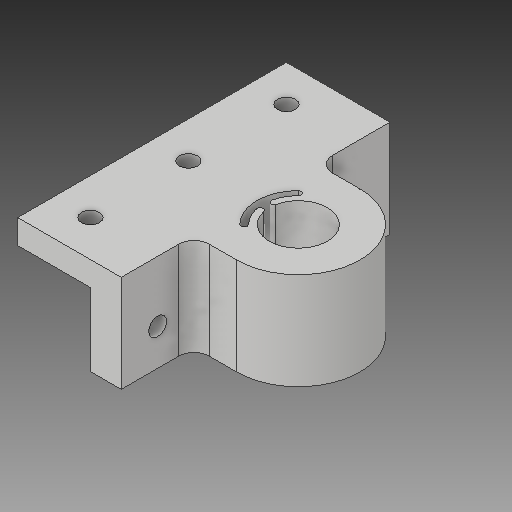
# Autodesk Inventor part: AxleBracket(3)
Saved by Autodesk Inventor 2018 (Build 220112000, 112)
## iProperties
Created: 2019-02-17
Part Number: AxleBracket(3)
Material: Generic
Document SubType Name: Modeling
Designer: anirudh
Density: 1 g/cm^3
Appearance: Default
Mass: 17.8737 g
Surface Area: 77.8022 cm^2
Volume: 17.8737 cm^3
Author: anirudh
Autodesk Inventor part; units mm, degrees
ref_plane "YZ Plane" through (0, 0, 0) normal (1, 0, 0) x (0, 1, 0)
ref_plane "XZ Plane" through (0, 0, 0) normal (0, 1, 0) x (-1, 0, 0)
ref_plane "XY Plane" through (0, 0, 0) normal (0, 0, 1) x (1, 0, 0)
sketch "Sketch1" plane through (0, 0, 0) normal (0, 1, 0) x (-1, 0, 0)
  arc A0 (0, 12.7) -> (0, -12.7) centre (0, 0) ccw
  line L0 (15.1638, 0) -> (15.1638, 12.7)
  line L1 (15.1638, 12.7) -> (15.1638, -12.7)
  line L2 (0, 12.7) -> (15.1638, 12.7)
  line L3 (0, -12.7) -> (15.1638, -12.7)
  arc A1 (6.0347, -6.0347) -> (6.0347, 6.0347) centre (0, 0) ccw
  arc A2 (5.8608, 1.285) -> (5.8669, -1.2566) centre (0, 0) ccw
  arc A3 (5.8608, 1.285) -> (5.8669, -1.2566) centre (0, 0) ccw
  arc A4 (5.8608, 1.285) -> (7.0867, 1.5971) centre (6.4884, 1.3835) ccw
  arc A5 (5.8608, 1.285) -> (7.0867, 1.5971) centre (6.4884, 1.3835) ccw
  arc A6 (7.0867, 1.5971) -> (5.1367, 5.1367) centre (0, 0) ccw
  arc A7 (6.0347, 6.0347) -> (5.1367, 5.1367) centre (5.5857, 5.5857) ccw
  arc A8 (6.0347, 6.0347) -> (5.1367, 5.1367) centre (5.5857, 5.5857) ccw
  arc A9 (5.1367, -5.1367) -> (6.0347, -6.0347) centre (5.5857, -5.5857) ccw
  arc A10 (5.1367, -5.1367) -> (6.0347, -6.0347) centre (5.5857, -5.5857) ccw
  arc A11 (7.0897, -1.5835) -> (5.8669, -1.2566) centre (6.4591, -1.4921) ccw
  arc A12 (7.0659, -1.6865) -> (5.8237, -1.444) centre (6.4591, -1.4921) ccw
  arc A13 (5.1367, -5.1367) -> (7.0897, -1.5835) centre (0, 0) ccw
  constraints: 36 point on circle, 14 centre point, 8 coincident, 8 end point, 2 perpendicular, 1 tangent
extrude "Extrusion1" add sketch "Sketch1" along normal blind 15
sketch "Sketch2" plane through (-15.1638, 0, 12.7) normal (0, 0, 1) x (1, 0, 0)
  line L0 (0, 15) -> (15.1638, 15) projected
  line L1 (15.1638, 0) -> (0, 0) projected
  line L2 (0, 15) -> (6.35, 15)
  line L3 (6.35, 15) -> (6.35, 0)
  line L4 (6.35, 0) -> (0, 0)
  line L5 (0, 0) -> (0, 15)
  dimension "d5" = 6.35
  constraints: 8 end point, 2 parallel, 1 horizontal, 1 perpendicular, 1 point on line
  measures "d5" distance of L3.end L4.end
extrude "Extrusion2" add sketch "Sketch2" along normal blind 15
sketch "Sketch3" plane through (0, 0, -12.7) normal (0, 0, -1) x (-1, 0, 0)
  line L0 (0, 15) -> (15.1638, 15) projected
  line L1 (15.1638, 0) -> (0, 0) projected
  line L2 (15.1638, 15) -> (8.8138, 15)
  line L3 (8.8138, 15) -> (8.8138, 0)
  line L4 (8.8138, 0) -> (15.1638, 0)
  line L5 (15.1638, 0) -> (15.1638, 15)
  dimension "d8" = 6.35
  constraints: 8 end point, 2 parallel, 1 horizontal, 1 perpendicular, 1 point on line
  measures "d8" distance of L4.end L3.end
extrude "Extrusion3" add sketch "Sketch3" along normal blind 15
sketch "Sketch4" plane through (-8.8138, 0, 12.7) normal (1, 0, 0) x (0, 0, -1)
  line L0 (-15, 15) -> (40.4, 15) projected
  line L1 (0, 0) -> (0, 15) projected
  line L2 (25.4, 15) -> (40.4, 15) projected
  line L3 (25.4, 0) -> (40.4, 0) projected
  line L4 (40.4, 0) -> (40.4, 15) projected
  line L5 (25.4, 0) -> (25.4, 15) projected
  circle A0 centre (-7.5, 7.5) radius 1.85
  circle A1 centre (32.9, 7.5) radius 1.85
  point P0 (12.7, 0)
  point P1 (-15, 0)
  dimension "d13" = 3.7
  dimension "d14" = 3.7
  constraints: 2 centre point
  measures "d13" diameter of A0
  measures "d14" diameter of A1
extrude "Extrusion4" cut sketch "Sketch4" against normal blind 15 contours A0 | A1
sketch "Sketch5" plane through (0, 15, 0) normal (0, 1, 0) x (1, 0, 0)
  line L0 (-8.8138, 12.7) -> (-8.8138, 27.7) projected
  line L1 (-15.1638, -27.7) -> (-8.8138, -27.7)
  line L2 (-8.8138, 27.7) -> (-15.1638, 27.7)
  line L3 (-8.8138, -12.7) -> (-8.8138, -27.7) projected
  line L4 (-8.8138, -27.7) -> (-8.8138, -12.7)
  arc A0 (0, -12.7) -> (0, 12.7) centre (0, 0) ccw projected
  line L5 (-8.8138, -12.7) -> (0, -12.7)
  line L6 (-8.8138, 27.7) -> (-8.8138, 12.7)
  line L7 (0, 12.7) -> (-8.8138, 12.7) projected
  line L8 (-8.8138, 12.7) -> (0, 12.7)
  arc A1 (0, -12.7) -> (0, 12.7) centre (0, 0) ccw
  arc A2 (-5.8752, -1.2175) -> (-5.8669, 1.2566) centre (0, 0) ccw
  arc A3 (-6.0347, -6.0347) -> (-5.1367, -5.1367) centre (-5.5857, -5.5857) ccw projected
  arc A4 (-6.0347, -6.0347) -> (-5.1367, -5.1367) centre (-5.5857, -5.5857) ccw
  arc A5 (-5.8608, -1.285) -> (-7.0867, -1.5971) centre (-6.4884, -1.3835) ccw projected
  arc A6 (-5.8608, -1.285) -> (-7.0867, -1.5971) centre (-6.4884, -1.3835) ccw
  arc A7 (-7.0897, 1.5835) -> (-5.8669, 1.2566) centre (-6.4591, 1.4921) ccw projected
  arc A8 (-7.0659, 1.6865) -> (-5.8237, 1.444) centre (-6.4591, 1.4921) ccw
  arc A9 (-5.1367, 5.1367) -> (-6.0347, 6.0347) centre (-5.5857, 5.5857) ccw projected
  arc A10 (-5.1367, 5.1367) -> (-6.0347, 6.0347) centre (-5.5857, 5.5857) ccw
  arc A11 (-7.0867, -1.5971) -> (-5.1367, -5.1367) centre (0, 0) ccw projected
  arc A12 (-6.0347, 6.0347) -> (-6.0347, -6.0347) centre (0, 0) ccw
  arc A13 (-5.1367, 5.1367) -> (-7.0897, 1.5835) centre (0, 0) ccw
  arc A14 (-7.1217, -1.4326) -> (-5.1367, -5.1367) centre (0, 0) ccw
  line L9 (-15.1638, -27.7) -> (-30.1638, -27.7)
  line L10 (-30.1638, -27.7) -> (-30.1638, 27.7)
  line L11 (-30.1638, 27.7) -> (-15.1638, 27.7)
  circle A15 centre (-22.6638, -20.2) radius 1.85
  circle A16 centre (-22.6638, 0) radius 1.85
  circle A17 centre (-22.6638, 20.2) radius 1.85
  dimension "d17" = 15
  dimension "d18" = 3.7
  dimension "d19" = 3.7
  dimension "d20" = 3.7
  constraints: 28 point on circle, 18 end point, 12 centre point, 8 coincident, 3 equal length, 3 perpendicular, 2 horizontal, 1 tangent, 1 vertical
  measures "d17" distance of L1.start L9.end
  measures "d18" diameter of A15
  measures "d19" diameter of A16
  measures "d20" diameter of A17
extrude "Extrusion5" add sketch "Sketch5" along normal blind 5 contours L7 A0 L5 L3 L1 L9 L10 L11 L2 L0 | A14 A5
fillet "Fillet1" radius 3.175 2 edges at (-8.8138, 10, 12.7) (-8.8138, 10, -12.7)
body "Solid1"
